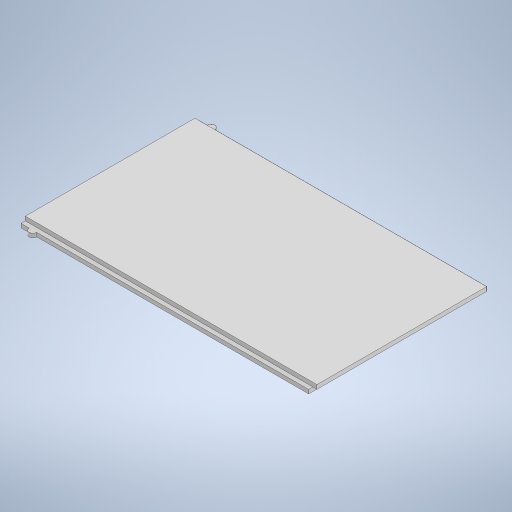
# Autodesk Inventor part: ControllerLid
Saved by Autodesk Inventor 2024 (Build 280153000, 153)
## iProperties
Created: 2024-03-27
Part Number: ControllerLid
Material: Generic
Document SubType Name: Modeling
Designer: bbbmi
Density: 1 g/cm^3
Appearance: Default
Author: bbbmi
Autodesk Inventor part; units mm, degrees
ref_plane "YZ Plane" through (0, 0, 0) normal (1, 0, 0) x (0, 1, 0)
ref_plane "XZ Plane" through (0, 0, 0) normal (0, 1, 0) x (-1, 0, 0)
ref_plane "XY Plane" through (0, 0, 0) normal (0, 0, 1) x (1, 0, 0)
sketch "Sketch1" plane through (0, 0, 0) normal (0, 1, 0) x (-1, 0, 0)
  line L0 (-36.727, -18.0642) -> (-36.727, 22.633)
  line L1 (-36.727, 22.633) -> (28.3668, 22.633)
  line L2 (28.3668, -18.0642) -> (-36.727, -18.0642)
  line L3 (30.2718, 23.5855) -> (28.3559, 23.5855)
  arc A0 (28.3559, 23.5855) -> (26.5779, 23.5855) centre (27.4669, 23.5855) ccw
  line L4 (26.5779, 23.5855) -> (-37.6795, 23.5855)
  line L5 (-37.6795, 23.5855) -> (-37.6795, -19.0167)
  line L6 (-37.6795, -19.0167) -> (26.5779, -19.0167)
  arc A1 (26.5779, -19.0167) -> (28.3559, -19.0167) centre (27.4669, -19.0167) ccw
  line L7 (28.3559, -19.0167) -> (30.2718, -19.0167)
  line L8 (30.2718, -18.6357) -> (27.8029, -18.6357)
  line L9 (27.1309, -18.6357) -> (-37.2985, -18.6357)
  line L10 (-37.2985, -18.6357) -> (-37.2985, 23.2045)
  line L11 (-37.2985, 23.2045) -> (27.1309, 23.2045)
  line L12 (27.8029, 23.2045) -> (30.2718, 23.2045)
  arc A2 (26.5779, -18.6357) -> (28.3559, -18.6357) centre (27.4669, -18.6524) ccw
  arc A3 (28.3559, 23.2045) -> (26.5779, 23.2045) centre (27.4669, 23.2045) ccw
  line L13 (30.2718, -18.6357) -> (30.2718, 23.2045)
  point P0 (0, 0)
  point P1 (25.8871, -17.6673)
  dimension "d0" = 0.381
  dimension "d1" = 0.889
  constraints: 28 end point, 8 point on circle, 4 centre point, 4 point on line, 2 other
  measures "d0" distance between parallel lines of L6 L9
  measures "d1" radius of A3
extrude "Extrusion1" add sketch "Sketch1" along normal blind 0.9144
sketch "Sketch2" plane through (0, 0.9144, 0) normal (0, 1, 0) x (1, 0, 0)
  line L0 (37.2985, 18.6357) -> (-26.5779, 18.6357) projected
  line L1 (-26.5779, -23.2045) -> (37.2985, -23.2045) projected
  line L2 (37.2985, 17.6451) -> (-26.5779, 17.6451)
  line L3 (-26.5779, -22.2139) -> (37.2985, -22.2139)
  line L4 (-26.5779, 17.6451) -> (-30.2718, 17.6451)
  line L5 (-30.2718, 18.6357) -> (-30.2718, -23.2045) projected
  line L6 (-26.5779, -22.2139) -> (-30.2718, -22.2139)
  line L7 (37.2985, 17.6451) -> (38.251, 17.6451)
  line L8 (38.251, 17.6451) -> (38.251, -22.2139)
  line L9 (38.251, -22.2139) -> (37.2985, -22.2139)
  point P0 (0, 0)
  dimension "d4" = 0.9906
  dimension "d5" = 0.9906
  dimension "d6" = 0.9525
  constraints: 14 end point, 3 parallel, 2 horizontal, 2 perpendicular, 2 point on line
  measures "d4" distance between parallel lines of L0 L2
  measures "d5" distance between parallel lines of L1 L3
  measures "d6" distance of L2.start L7.end
extrude "Extrusion2" add sketch "Sketch2" along normal blind 0.9652
body "Solid1"
